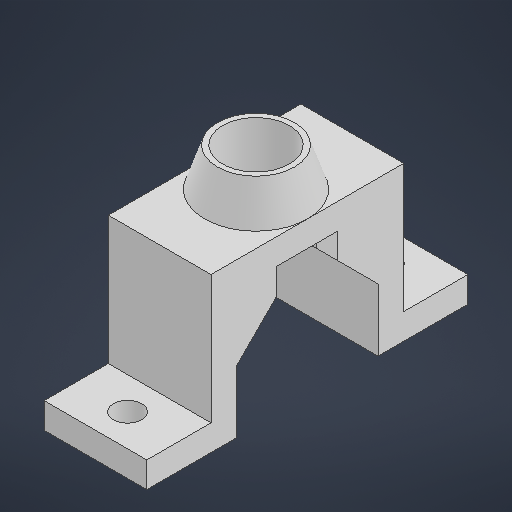
# Autodesk Inventor part: Bearing Mount
Saved by Autodesk Inventor 2025.1 (Build 291241000, 241)
## iProperties
Created: 2025-03-13
Part Number: Bearing Mount
Material: Generic
Document SubType Name: Modeling
Designer: jerem
Density: 1 g/cm^3
Appearance: Default
Author: jerem
## iProperties of the stored document Bearing Mount_3DPrint.ipt
Created: 2025-03-13
Part Number: Bearing Mount_3DPrint
Material: Generic
Document SubType Name: Modeling
Designer: jerem
Density: 1 g/cm^3
Appearance: Default
Author: jerem
Autodesk Inventor part; units mm, degrees
ref_plane "YZ Plane" through (0, 0, 0) normal (1, 0, 0) x (0, 1, 0)
ref_plane "XZ Plane" through (0, 0, 0) normal (0, 1, 0) x (-1, 0, 0)
ref_plane "XY Plane" through (0, 0, 0) normal (0, 0, 1) x (1, 0, 0)
sketch "Sketch1" plane through (0, 0, 0) normal (0, 1, 0) x (-1, 0, 0)
  line L0 (-4, -7.5) -> (4, -7.5)
  line L1 (4, -7.5) -> (4, 7.5)
  line L2 (4, 7.5) -> (-4, 7.5)
  line L3 (-4, 7.5) -> (-4, -7.5)
  line L4 (-4, -7.5) -> (4, 7.5) construction
  line L5 (4, -7.5) -> (-4, 7.5) construction
  line L6 (4, 7.5) -> (4, 12.5)
  line L7 (4, 12.5) -> (-4, 12.5)
  line L8 (-4, 12.5) -> (-4, 7.5)
  line L9 (-4, -7.5) -> (-4, -12.5)
  line L10 (-4, -12.5) -> (4, -12.5)
  line L11 (4, -12.5) -> (4, -7.5)
  circle A0 centre (0, 10) radius 1.1
  circle A1 centre (0, -10) radius 1.1
  line L12 (0, 10) -> (-4, 10) construction
  line L13 (0, -10) -> (-4, -10) construction
  line L14 (0, -10) -> (0, 0) construction
  line L15 (0, 0) -> (0, 10) construction
  line L16 (4, 5.5) -> (-4, 5.5)
  line L17 (4, -5.5) -> (-4, -5.5)
  circle A2 centre (0, 0) radius 2.6
  line L18 (-4.05, 2.3383) -> (0, 4.6765)
  line L19 (0, 4.6765) -> (4.05, 2.3383)
  line L20 (4.05, 2.3383) -> (4.05, -2.3383)
  line L21 (4.05, -2.3383) -> (0, -4.6765)
  line L22 (0, -4.6765) -> (-4.05, -2.3383)
  line L23 (-4.05, -2.3383) -> (-4.05, 2.3383)
  circle A3 centre (0, 0) radius 3
  point P0 (-4, -2.3671)
  point P1 (4, -2.3671)
  point P2 (4, 2.3671)
  point P3 (-4, 2.3671)
  dimension "d0" = 20
  dimension "d1" = 2.2
  dimension "d2" = 8
  dimension "d3" = 15
  dimension "d4" = 5
  dimension "d5" = 2
  dimension "d6" = 2
  dimension "d7" = 5.2
  dimension "d14" = 8.1
  dimension "d17" = 6
  constraints: 48 end point, 10 perpendicular, 4 centre point, 4 midpoint, 4 point on line, 3 coincident, 3 equal length, 2 collinear, 1 equal radius, 1 horizontal, 1 vertical, 13 other
  measures "d0" distance of L13.start L12.start
  measures "d1" diameter of A0
  measures "d2" distance of L6.end L7.end
  measures "d3" distance of L0.end L1.end
  measures "d4" distance of L1.end L6.end
  measures "d5" distance between parallel lines of L2 L16
  measures "d6" distance between parallel lines of L0 L17
  measures "d7" diameter of A2
  measures "d14" distance between parallel lines of L21 L18
  measures "d17" diameter of A3
extrude "Extrusion1" add sketch "Sketch1" against normal blind 2 contours L3 L17 L1 L0 | L0 L11 L10 L9 | L3 L2 L1 L16 | L8 L7 L6 L2
extrude "Extrusion2" add sketch "Sketch1" along normal blind 10 contours L3 L17 L1 L0 | L3 L2 L1 L16
extrude "Extrusion3" add sketch "Sketch1" against normal blind 2 from surface at 10 contours L3 L22 L21 L1 L17 | L3 L18 L19 L1 L21 L22 | L3 L16 L1 L19 L18 | A3
extrude "Extrusion4" add sketch "Sketch1" against normal blind 2 from surface at 8 contours L3 L22 L21 L1 L17 | L3 L16 L1 L19 L18
extrude "Extrusion5" add sketch "Sketch1" along normal blind 3 from surface at 10 contours A3
chamfer "Chamfer1" distance 1 distance2 3 1 edges at (3, 10, 0) measured on face at (3.5, 10, 0)
chamfer "Chamfer3" distance 3.13 angle 45 2 edges at (0, 6, 5.5) (0, 6, -5.5)
body "Solid1"
